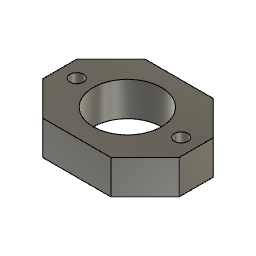
Pipe Break v1 v1 (Autodesk Fusion 360 design; units mm, degrees)
Autodesk Fusion 360 part; units mm, degrees
sketch "Sketch1" plane through (0, 0, 0) normal (0, 0, 1) x (1, 0, 0)
  line L0 (-50, 100) -> (50, 100)
  line L1 (50, 100) -> (100, 50)
  line L2 (100, 50) -> (100, 0)
  line L3 (100, 0) -> (50, -50)
  line L4 (50, -50) -> (-50, -50)
  line L5 (-50, -50) -> (-100, 0)
  line L6 (-100, 0) -> (-100, 50)
  line L7 (-100, 50) -> (-50, 100)
  constraint horizontal L0
  constraint perpendicular L0 L2
  constraint perpendicular L2 L4
  constraint perpendicular L4 L6
extrude "Extrude1" add sketch "Sketch1" along normal blind 50
hole "Hole1" at (-1.9643, 26.0412, 50) direction (0, 0, -1) diameter 100 depth 60 tip angle 118
hole "Hole2" at (76.0323, 27.1251, 50) direction (0, 0, -1) diameter 20 depth 60 tip angle 118
hole "Hole3" at (-75.8603, 25.7082, 50) direction (0, 0, -1) diameter 20 depth 60 tip angle 118
